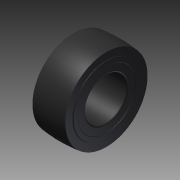
# Autodesk Inventor part: tire 16.2 od
Saved by Autodesk Inventor 2012 (Build 160160000, 160)
## iProperties
Created: 2011-11-26
Part Number: tire 16.2 od
Material: Default
Document SubType Name: Modeling
Designer: Antonella
Density: 1 g/cm^3
Author: Antonella
Autodesk Inventor part; units mm, degrees
ref_plane "YZ Plane" through (0, 0, 0) normal (1, 0, 0) x (0, 1, 0)
ref_plane "XZ Plane" through (0, 0, 0) normal (0, 1, 0) x (-1, 0, 0)
ref_plane "XY Plane" through (0, 0, 0) normal (0, 0, 1) x (1, 0, 0)
sketch "Sketch3" plane through (0, 0, 0) normal (0, 0, 1) x (1, 0, 0)
  line L0 (-112.014, 0) -> (112.014, 0) projected
  line L1 (0, -553.4025) -> (0, 332.2638) projected
  line L2 (-61.2196, 205.74) -> (61.2196, 205.74) construction
  line L3 (-80.01, 200.66) -> (80.01, 200.66) construction
  line L4 (-80.01, 101.6) -> (80.01, 101.6)
  line L5 (-80.01, 200.66) -> (-80.01, 101.6)
  line L6 (80.01, 200.66) -> (80.01, 101.6)
  arc A0 (80.01, 200.66) -> (-80.01, 200.66) centre (0, -426.8788) ccw
  point P0 (0, 0)
  point P1 (0, 205.74)
  point P2 (0, 200.66)
  dimension "d13" = 5.08
  dimension "d14" = 160.02
  dimension "d15" = 205.74
  dimension "d16" = 101.6
  constraints: 10 end point, 4 parallel, 3 point on circle, 2 midpoint, 2 perpendicular, 2 vertical alignment, 1 centre point
  measures "d13" distance between parallel lines of L2 L3
  measures "d14" distance of L3.start L3.end
  measures "d15" distance between parallel lines of L0 L2
  measures "d16" distance between parallel lines of L4 L0
revolve "Revolution1" add sketch "Sketch3" angle 360 about axis through (-10, 0, 0) along (1, 0, 0)
sketch "Sketch4" plane through (-80.01, 0, 0) normal (-1, 0, 0) x (0, 0, 1)
  circle A0 centre (0, 0) radius 101.6 projected
  circle A1 centre (0, 0) radius 139.7
  circle A2 centre (0, 0) radius 165.1
  dimension "d18" = 279.4
  dimension "d19" = 330.2
  constraints: 2 centre point, 2 coincident
  measures "d18" diameter of A1
  measures "d19" diameter of A2
extrude "Extrusion3" add sketch "Sketch4" along normal blind 2.54 contours A2
mirror "Mirror2" about plane through (0, 0, 0) normal (1, 0, 0) of "Extrusion3"
fillet "Fillet3" radius 3.175 4 edges at (-82.55, 0, -165.1) (-82.55, 0, -139.7) (82.55, 0, -139.7) (82.55, 0, -165.1)
fillet "Fillet4" radius 6.35 2 edges at (80.01, -101.6, 0) (-80.01, -101.6, 0)
body "Solid2"
